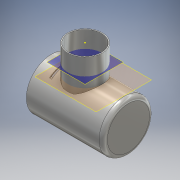
# Autodesk Inventor part: UR5 joint elbow2
Saved by Autodesk Inventor 2016 (Build 200138000, 138)
## iProperties
Created: 2017-12-24
Part Number: UR5 joint elbow2
Material: Aluminum 6061-AHC
Document SubType Name: Modeling
Designer: kornbot
Density: 2.7 g/cm^3
Appearance: Aluminum - Dark
Author: kornbot
Autodesk Inventor part; units mm, degrees
ref_plane "YZ Plane" through (0, 0, 0) normal (1, 0, 0) x (0, 1, 0)
ref_plane "XZ Plane" through (0, 0, 0) normal (0, 1, 0) x (-1, 0, 0)
ref_plane "XY Plane" through (0, 0, 0) normal (0, 0, 1) x (1, 0, 0)
sketch "Sketch1" plane through (0, 0, 0) normal (0, 0, 1) x (1, 0, 0)
  circle A0 centre (0, 0) radius 25.5
  circle A1 centre (0, 0) radius 27
  dimension "d0" = 51
  dimension "d1" = 54
  constraints: 2 centre point, 2 coincident
  measures "d0" diameter of A0
  measures "d1" diameter of A1
extrude "Extrusion1" add sketch "Sketch1" along normal blind 52
ref_plane "Work Plane1" through (0, 0, 26) normal (0, 0, -1) x (-1, 0, 0)
ref_plane "Work Plane2" through (0, 0, 26) normal (0, 0, -1) x (-1, 0, 0)
sketch "Sketch2" plane through (0, 0, 26) normal (0, 0, -1) x (-1, 0, 0)
  line L0 (30.9415, -24.1224) -> (27.5319, -24.1224)
  line L1 (27.5319, -24.1224) -> (27.5319, 25.1453)
  line L2 (27.5319, 25.1453) -> (30.9415, 25.1453)
  line L3 (30.9415, 25.1453) -> (30.9415, -24.1224)
  point P0 (0, 0)
  constraints: 8 end point, 2 parallel, 1 horizontal, 1 perpendicular
extrude "Extrusion2" add sketch "Sketch2" along normal blind 83.75
sketch "Sketch3" plane through (-30.9415, -24.1224, 26) normal (-1, 0, 0) x (0, 0, 1)
  line L0 (0, 0) -> (-83.75, 0) projected
  line L1 (0, 49.2677) -> (-83.75, 49.2677) projected
  line L2 (-83.75, 0) -> (-26, 0)
  line L3 (-26, 0) -> (-26, 49.2677)
  line L4 (-26, 49.2677) -> (-83.75, 49.2677)
  line L5 (-83.75, 49.2677) -> (-83.75, 0)
  line L6 (-83.75, 0) -> (-26, 49.2677)
  line L7 (-83.75, 49.2677) -> (-26, 0)
  circle A0 centre (-54.875, 24.6338) radius 39.1067
  circle A1 centre (-54.875, 24.6338) radius 37.5
  point P0 (-26, 24.1224)
  dimension "d6" = 75
  constraints: 12 end point, 2 centre point, 2 parallel, 1 coincident, 1 horizontal, 1 midpoint, 1 perpendicular, 1 point on line
  measures "d6" diameter of A1
extrude "Extrusion3" add sketch "Sketch3" against normal blind 86.25 contours A0 L1 A1 L5 L0 | L0 L3 A1 L1 A0
sketch "Sketch4" plane through (-30.9415, -24.1224, 26) normal (-1, 0, 0) x (0, 0, 1)
  line L0 (-26.6009, 49.2677) -> (-83.1491, 49.2677) projected
  line L1 (-83.0115, 0.207) -> (-26.6009, 49.2677)
  line L2 (-26.6009, 49.2677) -> (-83.1491, 49.2677)
  line L3 (-83.1491, 49.2677) -> (-26.6009, 0.7072)
  circle A0 centre (-54.875, 24.9874) radius 37.3287
  point P0 (-26, 24.1224)
  constraints: 6 end point, 1 centre point, 1 collinear, 1 midpoint
extrude "Extrusion4" cut sketch "Sketch4" against normal blind 147.5 contours L1 L3 L0 | A0
sketch "Sketch5" plane through (-30.9415, 25.1453, 26) normal (0, 1, 0) x (1, 0, 0)
  line L0 (3.4095, 0) -> (3.4095, 24.5021) projected
  line L1 (-0.8774, 24.5358) -> (3.4095, 24.5358)
  line L2 (3.4095, 24.5358) -> (3.4095, 0)
  line L3 (3.4095, 0) -> (-0.8774, 0)
  line L4 (-0.8774, 0) -> (-0.8774, 24.5358)
  point P0 (30.9415, 26)
  constraints: 8 end point, 2 parallel, 1 horizontal, 1 perpendicular
extrude "Extrusion5" cut sketch "Sketch5" against normal blind 83
ref_plane "Work Plane3" through (-30.9415, 0.5114, 10.2317) normal (0, 0, 1) x (1, 0, 0)
sketch "Sketch6" plane through (0, 0, 52) normal (0, 0, 1) x (1, 0, 0)
  circle A0 centre (0, 0) radius 25.5497
  constraints: 1 centre point, 1 coincident
extrude "Extrusion6" cut sketch "Sketch6" against normal blind 71.75
sketch "Sketch7" plane through (55.3085, 0.5114, -28.875) normal (1, 0, 0) x (0, 0, -1)
  circle A0 centre (0, 0) radius 39.1067
  point P0 (-28.875, -0.5114)
  constraints: 1 centre point
extrude "Extrusion7" add sketch "Sketch7" along normal blind 11.5
fillet "Fillet1" radius 6.5 1 edges at (66.8085, 0.5114, 10.2317)
sketch "Sketch8" plane through (-30.9415, 0.5114, -28.875) normal (-1, 0, 0) x (0, 0, 1)
  circle A0 centre (0, 0) radius 39.1067
  circle A1 centre (0, 0) radius 37.6591
  point P0 (28.875, -0.5114)
  constraints: 2 centre point, 1 coincident
extrude "Extrusion8" add sketch "Sketch8" along normal blind 21.5
sketch "Sketch9" plane through (-52.4415, 0.5114, -28.875) normal (-1, 0, 0) x (0, 0, 1)
  circle A0 centre (0, 0) radius 38.1825
  circle A1 centre (0, 0) radius 36.1825
  point P0 (28.875, -0.5114)
  dimension "d20" = 76.365
  dimension "d21" = 72.365
  constraints: 2 centre point, 1 coincident
  measures "d20" diameter of A0
  measures "d21" diameter of A1
extrude "Extrusion9" add sketch "Sketch9" against normal blind 4
sketch "Sketch10" plane through (0, 0, 52) normal (0, 0, 1) x (1, 0, 0)
  point P0 (0, 0)
body "Solid1"
